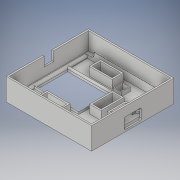
# Autodesk Inventor part: TOP
Saved by Autodesk Inventor 2019 (Build 230136000, 136)
## iProperties
Created: 2018-12-20
Part Number: TOP
Material: Типовые
Document SubType Name: Modeling
Designer: aldanstar
Density: 1 g/cm^3
Appearance: По умолчанию
Author: aldanstar
Autodesk Inventor part; units mm, degrees
ref_plane "YZ Plane" through (0, 0, 0) normal (1, 0, 0) x (0, 1, 0)
ref_plane "XZ Plane" through (0, 0, 0) normal (0, 1, 0) x (-1, 0, 0)
ref_plane "XY Plane" through (0, 0, 0) normal (0, 0, 1) x (1, 0, 0)
sketch "Эскиз1" plane through (0, 0, 0) normal (0, 1, 0) x (-1, 0, 0)
  line L0 (27.1, 26.1) -> (-27.1, 26.1)
  line L1 (-27.1, 26.1) -> (-27.1, -26.1)
  line L2 (-27.1, -26.1) -> (27.1, -26.1)
  line L3 (27.1, -26.1) -> (27.1, 26.1)
  line L4 (37.94, 0) -> (-37.94, 0) projected
  line L5 (0, -36.54) -> (0, 36.54) projected
  point P0 (0, 0)
  dimension "d0" = 54.2
  dimension "d1" = 52.2
  constraints: 8 end point, 2 parallel, 1 horizontal, 1 perpendicular, 2 other
  measures "d0" distance of L0.start L0.end
  measures "d1" distance of L0.end L1.end
extrude "Выдавливание1" add sketch "Эскиз1" along normal blind 14
shell "Оболочка1" thickness 1 removed faces 1 at (9.0333, 14, 8.7)
sketch "Эскиз2" plane through (27.1, 0, 26.1) normal (1, 0, 0) x (0, 0, -1)
  line L0 (22.2, 6.5) -> (30, 6.5) construction
  line L1 (30, 6.5) -> (30, 3) construction
  line L2 (30, 3) -> (22.2, 3) construction
  line L3 (22.2, 3) -> (22.2, 6.5) construction
  line L4 (0, 14) -> (52.2, 14) projected
  line L5 (26.1, -3) -> (26.1, 18) projected
  line L6 (30, 4.75) -> (22.2, 4.75) construction
  line L7 (20.6, 8.25) -> (31.6, 8.25)
  line L8 (31.6, 8.25) -> (31.6, 1.25)
  line L9 (31.6, 1.25) -> (20.6, 1.25)
  line L10 (20.6, 1.25) -> (20.6, 8.25)
  point P0 (26.1, 0)
  dimension "d5" = 7.5
  dimension "d6" = 7.8
  dimension "d7" = 3.5
  dimension "d114" = 7
  dimension "d115" = 11
  constraints: 18 end point, 4 parallel, 2 horizontal, 2 midpoint, 2 perpendicular, 3 other
  measures "d5" distance between parallel lines of L4 L0
  measures "d6" distance of L0.start L0.end
  measures "d7" distance of L0.end L1.end
  measures "d114" distance of L7.end L8.end
  measures "d115" distance of L7.start L7.end
extrude "Выдавливание2" cut sketch "Эскиз2" against normal up to surface (1 mm away)
sketch "Эскиз3" plane through (-26.1, 1, 25.1) normal (0, 1, 0) x (1, 0, 0)
  line L0 (43.8, 17) -> (49.7, 17) construction
  line L1 (49.7, 17) -> (49.7, 11.1) construction
  line L2 (49.7, 11.1) -> (43.8, 11.1) construction
  line L3 (43.8, 11.1) -> (43.8, 17) construction
  line L4 (52.2, 50.2) -> (52.2, 0) construction
  line L5 (52.2, 0) -> (0, 0) construction
  line L6 (46.75, 17) -> (46.75, 11.1) construction
  line L7 (49.7, 14.05) -> (43.8, 14.05) construction
  circle A0 centre (46.75, 14.05) radius 1.75
  point P0 (26.1, 25.1)
  dimension "d11" = 5.9
  dimension "d12" = 5.9
  dimension "d15" = 3.5
  dimension "d18" = 17
  dimension "d19" = 2.5
  constraints: 12 end point, 5 midpoint, 2 parallel, 1 centre point, 1 horizontal, 1 perpendicular
  measures "d11" distance of L0.start L0.end
  measures "d12" distance of L0.end L1.end
  measures "d15" diameter of A0
  measures "d18" distance between parallel lines of L0 L5
  measures "d19" distance from line of L7.start L4
extrude "Выдавливание3" cut sketch "Эскиз3" against normal through all
mirror "Зеркальное отражение2" about plane through (0, 0, 0) normal (0, 0, 1) of "Выдавливание3"
sketch "Эскиз4" plane through (-26.1, 1, 25.1) normal (0, 1, 0) x (1, 0, 0)
  line L0 (30.1, 9.9) -> (35.85, 9.9) construction
  line L1 (35.85, 9.9) -> (35.85, 4.15) construction
  line L2 (35.85, 4.15) -> (30.1, 4.15) construction
  line L3 (30.1, 4.15) -> (30.1, 9.9) construction
  line L4 (0, 0) -> (52.2, 0) construction
  line L5 (52.2, 0) -> (52.2, 50.2) construction
  line L6 (37.225, 11.275) -> (28.725, 11.275)
  line L7 (28.725, 11.275) -> (28.725, 2.775)
  line L8 (28.725, 2.775) -> (37.225, 2.775)
  line L9 (37.225, 2.775) -> (37.225, 11.275)
  line L10 (35.85, 7.025) -> (30.1, 7.025) construction
  line L11 (32.975, 9.9) -> (32.975, 4.15) construction
  line L12 (25.8, 44.7) -> (13.2, 44.7)
  line L13 (13.2, 44.7) -> (13.2, 39.4)
  line L14 (13.2, 39.4) -> (25.8, 39.4)
  line L15 (25.8, 39.4) -> (25.8, 44.7)
  line L16 (53.2, 51.2) -> (-1, 51.2) construction
  line L17 (0, 50.2) -> (52.2, 50.2) projected
  line L18 (0, 0) -> (0, 50.2) projected
  line L19 (39.4, 31.4) -> (34.1, 31.4)
  line L20 (34.1, 31.4) -> (34.1, 18.8)
  line L21 (34.1, 18.8) -> (39.4, 18.8)
  line L22 (39.4, 18.8) -> (39.4, 31.4)
  line L23 (-11.84, 25.1) -> (64.04, 25.1) projected
  point P0 (26.1, 25.1)
  dimension "d20" = 5.75
  dimension "d21" = 9.9
  dimension "d22" = 22.1
  dimension "d23" = 8.5
  dimension "d26" = 12.6
  dimension "d27" = 5.3
  dimension "d29" = 10.8
  dimension "d30" = 25.8
  dimension "d31" = 5.3
  dimension "d32" = 12.6
  dimension "d33" = 18.1
  constraints: 36 end point, 8 parallel, 6 perpendicular, 4 horizontal, 4 midpoint, 3 other
  measures "d20" distance of L0.end L1.end
  measures "d21" distance between parallel lines of L0 L4
  measures "d22" distance between parallel lines of L5 L3
  measures "d23" distance of L8.end L6.start
  measures "d26" distance of L14.end L13.end
  measures "d27" distance of L14.end L12.start
  measures "d29" distance between parallel lines of L17 L14
  measures "d30" distance between parallel lines of L18 L15
  measures "d31" distance of L19.start L19.end
  measures "d32" distance of L21.end L19.start
  measures "d33" distance between parallel lines of L5 L20
extrude "Выдавливание4" cut sketch "Эскиз4" against normal through all contours L9 L8 L7 L6
extrude "Выдавливание5" cut sketch "Эскиз4" against normal through all contours L15 L14 L13 L12
mirror "Зеркальное отражение3" about plane through (0, 0, 0) normal (0, 0, 1) of "Выдавливание5"
extrude "Выдавливание6" cut sketch "Эскиз4" against normal through all contours L22 L23 L20 L19 | L22 L21 L20 L23
sketch "Эскиз5" plane through (-26.1, 1, 25.1) normal (0, 1, 0) x (1, 0, 0)
  line L0 (42.8, 28.9) -> (44.8, 28.9) construction
  line L1 (44.8, 28.9) -> (44.8, 21.3)
  line L2 (44.8, 21.3) -> (42.8, 21.3) construction
  line L3 (42.8, 21.3) -> (42.8, 28.9)
  line L4 (52.2, 0) -> (52.2, 50.2) projected
  line L5 (-11.84, 25.1) -> (64.04, 25.1) projected
  line L6 (42.8, 21.3) -> (44.8, 21.3) construction
  line L7 (49.2, 21.3) -> (49.2, 19.3)
  line L8 (49.2, 19.3) -> (42.8, 19.3)
  line L9 (42.8, 19.3) -> (42.8, 21.3)
  line L10 (44.8, 21.3) -> (49.2, 21.3)
  line L11 (42.8, 28.9) -> (44.8, 28.9) construction
  line L12 (49.2, 28.9) -> (49.2, 30.9)
  line L13 (49.2, 30.9) -> (42.8, 30.9)
  line L14 (42.8, 30.9) -> (42.8, 28.9)
  line L15 (44.8, 28.9) -> (49.2, 28.9)
  point P0 (26.1, 25.1)
  dimension "d39" = 2
  dimension "d40" = 7.4
  dimension "d41" = 7.6
  dimension "d42" = 6.4
  dimension "d43" = 2
  constraints: 28 end point, 8 parallel, 5 horizontal, 5 perpendicular, 2 equal length, 1 other
  measures "d39" distance of L1.end L2.end
  measures "d40" distance between parallel lines of L4 L1
  measures "d41" distance between parallel lines of L0 L2
  measures "d42" distance of L7.end L8.end
  measures "d43" distance of L7.start L7.end
extrude "Выдавливание7" add sketch "Эскиз5" along normal blind 5.4
fillet "Сопряжение2" radius 1 3 edges at (20.9, 6.4, 3.8) (20.9, 6.4, -3.8) (18.7, 6.4, 0)
sketch "Эскиз6" plane through (0, 0, 0) normal (0, -1, 0) x (1, 0, 0)
  line L0 (-24.1, -10) -> (2.9, -10)
  line L1 (2.9, -10) -> (2.9, 10)
  line L2 (2.9, 10) -> (-24.1, 10)
  line L3 (-24.1, 10) -> (-24.1, -10)
  line L4 (-26.1, -25.1) -> (-26.1, 25.1) projected
  line L5 (-37.94, 0) -> (37.94, 0) projected
  point P0 (0, 0)
  dimension "d47" = 29
  dimension "d48" = 20
  dimension "d118" = 2
  constraints: 8 end point, 2 parallel, 1 horizontal, 1 perpendicular, 1 other
  measures "d47" distance between parallel lines of L4 L1
  measures "d48" distance between parallel lines of L0 L2
  measures "d118" distance between parallel lines of L4 L3
extrude "Выдавливание8" cut sketch "Эскиз6" against normal up to surface (1 mm away)
sketch "Эскиз10" plane through (-26.1, 1, 25.1) normal (0, 1, 0) x (1, 0, 0)
  line L0 (0, 0) -> (52.2, 0) projected
  line L1 (52.2, 50.2) -> (0, 50.2) projected
  line L2 (52.2, 0) -> (0, 0) projected
  line L3 (52.2, 0) -> (52.2, 8)
  line L4 (52.2, 50.2) -> (52.2, 42.2)
  line L5 (52.2, 42.2) -> (50.2, 42.2) construction
  line L6 (50.2, 47.7) -> (2, 47.7)
  line L7 (50.2, 47.7) -> (50.2, 42.2)
  line L8 (50.2, 2.5) -> (2, 2.5)
  line L9 (50.2, 2.5) -> (50.2, 8)
  line L10 (50.2, 8) -> (52.2, 8) construction
  line L11 (2, 2.5) -> (2, 47.7)
  line L12 (50.2, 8) -> (50.2, 19.3)
  line L13 (52.2, 42.2) -> (52.2, 8)
  line L14 (53.2, -1) -> (53.2, 51.2) projected
  line L15 (49.2, 29.9) -> (49.2, 28.9) projected
  line L16 (49.2, 29.9) -> (49.2, 30.9) projected
  line L17 (44.8, 28.9) -> (49.2, 28.9) projected
  line L18 (44.8, 21.3) -> (44.8, 28.9) projected
  line L19 (49.2, 21.3) -> (44.8, 21.3) projected
  line L20 (49.2, 21.3) -> (49.2, 20.3) projected
  line L21 (49.2, 19.3) -> (49.2, 20.3) projected
  line L22 (49.2, 19.3) -> (50.2, 19.3)
  line L23 (49.2, 30.9) -> (50.2, 30.9)
  line L24 (50.2, 19.3) -> (50.2, 30.9) construction
  line L25 (50.2, 30.9) -> (50.2, 42.2)
  line L26 (0, 0) -> (0, 50.2)
  point P0 (26.1, 25.1)
  dimension "d66" = 8
  dimension "d67" = 2
  dimension "d68" = 2.5
  dimension "d69" = 2.5
  dimension "d70" = 2
  dimension "d117" = 2
  constraints: 32 end point, 7 perpendicular, 4 vertical, 3 parallel, 1 collinear, 1 horizontal, 1 point on line
  measures "d66" distance of L1.start L4.end
  measures "d67" distance of L4.end L5.end
  measures "d68" distance between parallel lines of L1 L6
  measures "d69" distance between parallel lines of L2 L8
  measures "d70" distance between parallel lines of L3 L9
  measures "d117" distance between parallel lines of L26 L11
extrude "Выдавливание12" add sketch "Эскиз10" along normal blind 1.9
sketch "Эскиз11" plane through (-26.1, 2.9, 25.1) normal (0, 1, 0) x (1, 0, 0)
  line L0 (50.2, 47.7) -> (2, 47.7) projected
  line L1 (46.1, 47.7) -> (6.1, 47.7)
  line L2 (6.1, 47.7) -> (6.1, 48.8)
  line L3 (6.1, 48.8) -> (46.1, 48.8)
  line L4 (46.1, 48.8) -> (46.1, 47.7)
  line L5 (0, 50.2) -> (52.2, 50.2) projected
  line L6 (26.1, 61.64) -> (26.1, -11.44) projected
  point P0 (26.1, 25.1)
  dimension "d73" = 1.4
  dimension "d74" = 40
  constraints: 8 end point, 2 parallel, 1 horizontal, 1 perpendicular, 1 point on line, 1 other
  measures "d73" distance between parallel lines of L5 L3
  measures "d74" distance between parallel lines of L4 L2
extrude "Выдавливание13" add sketch "Эскиз11" along normal up to surface (3.5 mm away)
mirror "Зеркальное отражение4" about plane through (0, 0, 0) normal (0, 0, 1) of "Выдавливание13"
fillet "Сопряжение6" radius 2 4 edges at (20, 2.9, -23.15) (-20, 2.9, -23.15) (-20, 2.9, 23.15) (20, 2.9, 23.15)
fillet "Сопряжение6" radius 1 6 edges at (0, 6.4, -23.7) (0, 6.4, 23.7) (26.6, 1.25, 5.5) (26.6, 8.25, 5.5) (26.6, 8.25, -5.5) (26.6, 1.25, -5.5)
sketch "Эскиз12" plane through (-24.1, 1, -11.1737) normal (0, 1, 0) x (1, 0, 0)
  line L0 (37.4, -17.4737) -> (32.1, -17.4737)
  line L1 (37.4, -4.8737) -> (37.4, -17.4737)
  line L2 (32.1, -4.8737) -> (37.4, -4.8737)
  line L3 (32.1, -17.4737) -> (32.1, -4.8737)
  line L4 (23.8, 3.1263) -> (11.2, 3.1263)
  line L5 (23.8, 8.4263) -> (23.8, 3.1263)
  line L6 (11.2, 8.4263) -> (23.8, 8.4263)
  line L7 (11.2, 3.1263) -> (11.2, 8.4263)
  line L8 (11.2, -30.7737) -> (11.2, -25.4737)
  line L9 (23.8, -30.7737) -> (11.2, -30.7737)
  line L10 (23.8, -25.4737) -> (23.8, -30.7737)
  line L11 (11.2, -25.4737) -> (23.8, -25.4737)
  line L12 (24.8, 2.1263) -> (10.2, 2.1263)
  line L13 (10.2, 2.1263) -> (10.2, 9.4263)
  line L14 (10.2, 9.4263) -> (24.8, 9.4263)
  line L15 (24.8, 9.4263) -> (24.8, 2.1263)
  line L16 (31.1, -18.4737) -> (38.4, -18.4737)
  line L17 (38.4, -18.4737) -> (38.4, -3.8737)
  line L18 (38.4, -3.8737) -> (31.1, -3.8737)
  line L19 (31.1, -3.8737) -> (31.1, -18.4737)
  line L20 (24.8, -31.7737) -> (10.2, -31.7737)
  line L21 (10.2, -31.7737) -> (10.2, -24.4737)
  line L22 (10.2, -24.4737) -> (24.8, -24.4737)
  line L23 (24.8, -24.4737) -> (24.8, -31.7737)
  line L24 (23.8, 3.1263) -> (11.2, 3.1263) projected
  line L25 (11.2, 3.1263) -> (11.2, 8.4263) projected
  line L26 (11.2, 8.4263) -> (23.8, 8.4263) projected
  line L27 (23.8, 8.4263) -> (23.8, 3.1263) projected
  line L28 (32.1, -4.8737) -> (37.4, -4.8737) projected
  line L29 (32.1, -17.4737) -> (32.1, -4.8737) projected
  line L30 (37.4, -17.4737) -> (32.1, -17.4737) projected
  line L31 (37.4, -4.8737) -> (37.4, -17.4737) projected
  line L32 (11.2, -25.4737) -> (23.8, -25.4737) projected
  line L33 (11.2, -30.7737) -> (11.2, -25.4737) projected
  line L34 (23.8, -30.7737) -> (11.2, -30.7737) projected
  line L35 (23.8, -25.4737) -> (23.8, -30.7737) projected
  point P0 (24.1, -11.1737)
  dimension "d79" = 1
  dimension "d80" = 1
  dimension "d81" = 1
  constraints: 48 end point, 12 collinear, 9 other
  measures "d79" distance between parallel lines of L5 L15
  measures "d80" distance between parallel lines of L0 L16
  measures "d81" distance between parallel lines of L10 L23
extrude "Выдавливание14" add sketch "Эскиз12" along normal up to surface (5.4 mm away)
sketch "Эскиз13" plane through (-24.1, 1, -11.1737) normal (0, 1, 0) x (1, 0, 0)
  line L0 (36.4, -31.7987) -> (39.4, -31.7987)
  line L1 (39.4, -31.7987) -> (39.4, -26.6987)
  line L2 (39.4, -26.6987) -> (36.4, -26.6987)
  line L3 (36.4, -26.6987) -> (36.4, -31.7987)
  line L4 (26.725, -24.9987) -> (26.725, -33.4987) construction
  line L5 (26.725, -29.2487) -> (35.225, -29.2487) construction
  line L6 (35.225, -33.4987) -> (35.225, -24.9987) construction
  line L7 (37.9, -31.7987) -> (37.9, -26.6987) construction
  line L8 (50.2, 13.9263) -> (50.2, -36.2737) construction
  line L9 (31.2, 1.4263) -> (27.2, 1.4263)
  line L10 (27.2, 1.4263) -> (27.2, 6.4263)
  line L11 (27.2, 6.4263) -> (31.2, 6.4263)
  line L12 (31.2, 6.4263) -> (31.2, 1.4263)
  line L13 (29.2, 1.4263) -> (29.2, 6.4263) construction
  line L14 (31.2, 3.9263) -> (27.2, 3.9263) construction
  line L15 (-2, 13.9263) -> (50.2, 13.9263) construction
  line L16 (26.725, -33.4987) -> (26.725, -24.9987) projected
  line L17 (35.225, -24.9987) -> (35.225, -33.4987) projected
  line L18 (50.2, 13.9263) -> (50.2, -5.6737) projected
  line L19 (-2, 13.9263) -> (50.2, 13.9263) projected
  dimension "d68" = 2.5
  dimension "d85" = 5.1
  dimension "d86" = 12.3
  dimension "d87" = 3
  dimension "d88" = 21
  dimension "d89" = 4
  dimension "d90" = 5
  dimension "d91" = 10
  constraints: 32 end point, 8 midpoint, 4 collinear, 4 parallel, 2 horizontal, 2 perpendicular, 1 other
  measures "d85" distance of L0.end L1.end
  measures "d86" distance between parallel lines of L8 L7
  measures "d87" distance between parallel lines of L1 L3
  measures "d88" distance between parallel lines of L8 L13
  measures "d89" distance of L10.end L11.end
  measures "d90" distance of L11.end L9.start
  measures "d91" distance between parallel lines of L15 L14
extrude "Выдавливание15" cut sketch "Эскиз13" against normal through all
sketch "Эскиз14" plane through (-24.1, 1, -11.1737) normal (0, 1, 0) x (1, 0, 0)
  line L0 (31.2, 1.4263) -> (27.2, 1.4263)
  line L1 (31.2, 6.4263) -> (31.2, 1.4263)
  line L2 (27.2, 6.4263) -> (31.2, 6.4263)
  line L3 (27.2, 1.4263) -> (27.2, 6.4263)
  line L4 (26.7, 0.9263) -> (31.7, 0.9263)
  line L5 (31.7, 0.9263) -> (31.7, 6.9263)
  line L6 (31.7, 6.9263) -> (26.7, 6.9263)
  line L7 (26.7, 6.9263) -> (26.7, 0.9263)
  line L8 (36.4, -31.7987) -> (36.4, -26.6987)
  line L9 (36.4, -26.6987) -> (39.4, -26.6987)
  line L10 (39.4, -26.6987) -> (39.4, -31.7987)
  line L11 (39.4, -31.7987) -> (36.4, -31.7987)
  line L12 (35.9, -26.1987) -> (35.9, -32.2987)
  line L13 (35.9, -32.2987) -> (39.9, -32.2987)
  line L14 (39.9, -32.2987) -> (39.9, -26.1987)
  line L15 (39.9, -26.1987) -> (35.9, -26.1987)
  line L16 (39.4, -26.6987) -> (39.4, -31.7987) projected
  line L17 (36.4, -26.6987) -> (39.4, -26.6987) projected
  line L18 (36.4, -31.7987) -> (36.4, -26.6987) projected
  line L19 (39.4, -31.7987) -> (36.4, -31.7987) projected
  line L20 (31.2, 6.4263) -> (31.2, 1.4263) projected
  line L21 (27.2, 6.4263) -> (31.2, 6.4263) projected
  line L22 (27.2, 1.4263) -> (27.2, 6.4263) projected
  line L23 (31.2, 1.4263) -> (27.2, 1.4263) projected
  dimension "d94" = 0.5
  dimension "d116" = 0.5
  constraints: 32 end point, 8 collinear, 6 other
  measures "d94" distance between parallel lines of L0 L4
  measures "d116" distance between parallel lines of L8 L12
extrude "Выдавливание16" add sketch "Эскиз14" along normal blind 2.5
sketch "Эскиз16" plane through (-27.1, 0, 26.1) normal (-1, 0, 0) x (0, 0, 1)
  line L0 (-29.1, 14) -> (-23.1, 14)
  line L1 (-23.1, 14) -> (-23.1, 8)
  line L2 (-23.1, 8) -> (-29.1, 8)
  line L3 (-29.1, 8) -> (-29.1, 14)
  line L4 (-26.1, -2.8) -> (-26.1, 16.8) projected
  line L5 (-52.2, 14) -> (0, 14) projected
  point P0 (-26.1, 0)
  dimension "d111" = 6
  constraints: 8 end point, 2 parallel, 2 perpendicular, 1 collinear, 1 horizontal, 1 other
  measures "d111" distance of L2.end L0.start
extrude "Выдавливание18" cut sketch "Эскиз16" against normal up to surface (1 mm away)
sketch "Эскиз17" plane through (16.7, 1, 5.8) normal (0, 1, 0) x (1, 0, 0)
  line L0 (-40.8, -16.8) -> (-40.8, 28.4) projected
  line L1 (-12.8, -5.2) -> (-40.8, -5.2)
  line L2 (-40.8, -5.2) -> (-40.8, 16.8)
  line L3 (-40.8, 16.8) -> (-12.8, 16.8)
  line L4 (-12.8, 16.8) -> (-12.8, -5.2)
  line L5 (-13.8, -4.2) -> (-40.8, -4.2) projected
  line L6 (-13.8, 15.8) -> (-13.8, -4.2) projected
  line L7 (-40.8, 15.8) -> (-13.8, 15.8) projected
  point P0 (-16.7, 5.8)
  dimension "d119" = 1
  dimension "d120" = 1
  dimension "d121" = 1
  constraints: 8 end point, 2 parallel, 1 horizontal, 1 perpendicular, 1 point on line
  measures "d119" distance between parallel lines of L1 L5
  measures "d120" distance between parallel lines of L4 L6
  measures "d121" distance between parallel lines of L7 L3
extrude "Выдавливание19" add sketch "Эскиз17" along normal blind 1.5 contours L0 L5 L6 L7 L3 L4 L1
fillet "Сопряжение8" radius 1.5 1 edges at (-24.1, 2.9, 0)
fillet "Сопряжение9" radius 1 3 edges at (-10.8401, 2.5, -10) (2.9, 2.5, 0) (-10.8401, 2.5, 10)
